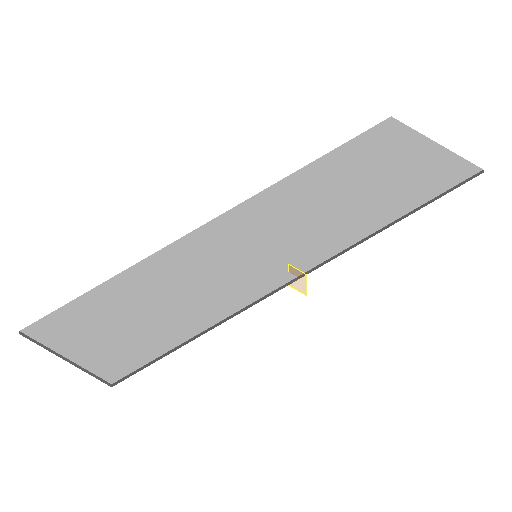
# Autodesk Inventor part: outlet strip
Saved by Autodesk Inventor 2022 (Build 260148000, 148)
## iProperties
Created: 2007-05-11
Part Number: outlet strip
Material: Steel, Mild
Document SubType Name: Modeling
Designer: LionelF
Density: 7.86 g/cm^3
Mass: 1241.48 g
Surface Area: 1030.44 cm^2
Volume: 157.95 cm^3
Appearance: Steel
Author: LionelF
Autodesk Inventor part; units mm, degrees
ref_plane "YZ Plane" through (0, 0, 0) normal (1, 0, 0) x (0, 1, 0)
ref_plane "XZ Plane" through (0, 0, 0) normal (0, 1, 0) x (-1, 0, 0)
ref_plane "XY Plane" through (0, 0, 0) normal (0, 0, 1) x (1, 0, 0)
sketch "Sketch1" plane through (0, 0, 0) normal (0, 0, 1) x (1, 0, 0)
  line L0 (1.6497, -1.7353) -> (112.7747, -1.7353)
  line L1 (112.7747, -1.7353) -> (112.7747, 1.4397)
  line L2 (112.7747, 1.4397) -> (1.6497, 1.4397)
  line L3 (1.6497, 1.4397) -> (1.6497, -1.7353)
  dimension "d0" = 111.125
  dimension "d1" = 3.175
  constraints: 8 end point, 2 parallel, 1 horizontal, 1 perpendicular
  measures "d0" distance of L1.end L2.end
  measures "d1" distance of L2.end L0.start
extrude "Extrusion1" add sketch "Sketch1" along normal blind 447.675
ref_plane "Work Plane1" through (112.7747, -1.7353, 223.8375) normal (0, 0, 1) x (1, 0, 0)
body "Solid1"
